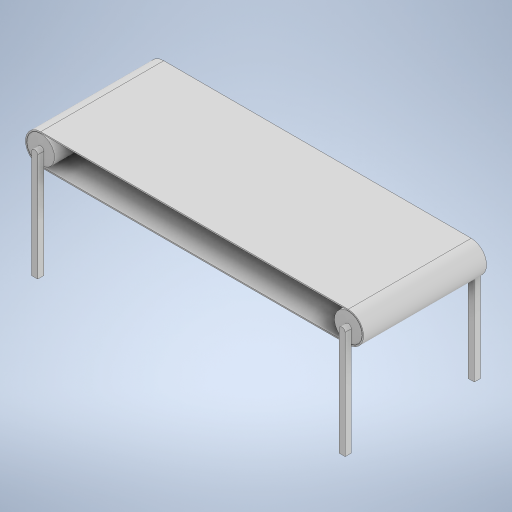
# Autodesk Inventor part: Banda
Saved by Autodesk Inventor 2023 (Build 270158000, 158)
## iProperties
Created: 2023-06-01
Part Number: Banda
Material: Generic
Document SubType Name: Modeling
Designer: Zenbook
Density: 1 g/cm^3
Appearance: Default
Author: Zenbook
Autodesk Inventor part; units mm, degrees
ref_plane "YZ Plane" through (0, 0, 0) normal (1, 0, 0) x (0, 1, 0)
ref_plane "XZ Plane" through (0, 0, 0) normal (0, 1, 0) x (-1, 0, 0)
ref_plane "XY Plane" through (0, 0, 0) normal (0, 0, 1) x (1, 0, 0)
sketch "Sketch1" plane through (0, 0, 0) normal (0, 0, 1) x (1, 0, 0)
  arc A0 (0, 25) -> (0, -25) centre (0, 0) ccw
  arc A1 (500, -25) -> (500, 25) centre (500, 0) ccw
  line L0 (0, 25) -> (500, 25)
  line L1 (500, -25) -> (0, -25)
  arc A2 (0, 23) -> (0, -23) centre (0, 0) ccw
  arc A3 (500, -23) -> (500, 23) centre (500, 0) ccw
  line L2 (500, 0) -> (500, 23) construction
  line L3 (500, 0) -> (523, 0) construction
  line L4 (0, 23) -> (500, 23)
  line L5 (0, -23) -> (500, -23)
  dimension "D" = 50
  dimension "d2" = 50
  dimension "r" = 23
  dimension "d6" = 23
  dimension "d7" = 90
  dimension "L" = 500
  constraints: 12 end point, 9 point on circle, 4 centre point, 4 tangent, 3 coincident, 1 horizontal, 1 parallel, 1 perpendicular
  measures "D" diameter of A0
  measures "d2" diameter of A1
  measures "r" radius of A2
  measures "d6" radius of A3
  measures "d7" angle of L3 L2
  measures "L" distance of A1.centre point (0, 0)
extrude "Extrusion1" add sketch "Sketch1" against normal blind 200
sketch "Sketch2" plane through (0, 0, 0) normal (0, 0, 1) x (1, 0, 0)
  circle A0 centre (0, 0) radius 22.5
  arc A1 (500, -23) -> (500, 23) centre (500, 0) ccw construction
  circle A2 centre (500, 0) radius 22.5
  point P0 (300, -23)
  dimension "d" = 45
  dimension "d12" = 45
  constraints: 2 centre point, 2 coincident
  measures "d" diameter of A0
  measures "d12" diameter of A2
extrude "Extrusion2" add sketch "Sketch2" against normal blind 200
sketch "Sketch3" plane through (0, 0, 0) normal (0, 0, 1) x (1, 0, 0)
  arc A0 (5, 0) -> (-5, 0) centre (0, 0) ccw
  circle A1 centre (500, 0) radius 22.5 construction
  arc A2 (505, 0) -> (495, 0) centre (500, 0) ccw
  line L0 (5, 0) -> (5, -175)
  line L1 (5, -175) -> (-5, -175)
  line L2 (-5, -175) -> (-5, 0)
  line L3 (495, 0) -> (495, -175)
  line L4 (495, -175) -> (505, -175)
  line L5 (505, -175) -> (505, 0)
  dimension "altura" = 175
  dimension "d19" = 175
  dimension "d20" = 5
  dimension "d21" = 5
  constraints: 12 end point, 4 point on circle, 2 centre point, 2 coincident, 2 parallel
  measures "altura" distance of L0.start L0.end
  measures "d19" distance of L3.end L3.start
  measures "d20" radius of A0
  measures "d21" radius of A2
extrude "Extrusion3" add sketch "Sketch3" along normal blind 10
sketch "Sketch4" plane through (0, 0, -200) normal (0, 0, -1) x (-1, 0, 0)
  arc A0 (5, 0) -> (-5, 0) centre (0, 0) ccw projected
  arc A1 (5, 0) -> (-5, 0) centre (0, 0) ccw
  arc A2 (-495, 0) -> (-505, 0) centre (-500, 0) ccw projected
  arc A3 (-495, 0) -> (-505, 0) centre (-500, 0) ccw
  line L0 (-505, -175) -> (-505, 0) projected
  line L1 (-495, 0) -> (-495, -175) projected
  line L2 (-495, 0) -> (-495, -175)
  line L3 (-495, -175) -> (-505, -175)
  line L4 (-505, -175) -> (-505, 0)
  line L5 (5, -175) -> (-5, -175) projected
  line L6 (-5, 0) -> (-5, -175)
  line L7 (-5, -175) -> (5, -175)
  line L8 (5, -175) -> (5, 0)
  point P0 (-5, 0)
  constraints: 12 end point, 4 point on circle, 2 centre point, 2 coincident, 2 parallel
extrude "Extrusion4" add sketch "Sketch4" along normal blind 10
equation "\"d2\" = D"
equation "\"d6\" = r"
equation "\"d12\" = d"
equation "\"d19\" = altura"
body "Solid1"
